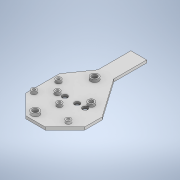
# Autodesk Inventor part: Część1
Saved by Autodesk Inventor 2020 (Build 240168000, 168)
## iProperties
Created: 2019-04-24
Part Number: Część1
Material: Ogólny
Document SubType Name: Modeling
Designer: atmat
Density: 1 g/cm^3
Appearance: Domyślna
Author: atmat
Autodesk Inventor part; units mm, degrees
ref_plane "YZ Plane" through (0, 0, 0) normal (1, 0, 0) x (0, 1, 0)
ref_plane "XZ Plane" through (0, 0, 0) normal (0, 1, 0) x (-1, 0, 0)
sketch "Szkic1" plane through (0, 0, 0) normal (0, 1, 0) x (-1, 0, 0)
  circle A0 centre (0, 22.5) radius 2
  circle A1 centre (0, -22.5) radius 2
  circle A2 centre (0, 22.5) radius 11.25 construction
  circle A3 centre (0, -22.5) radius 11.25 construction
  circle A4 centre (0, 0) radius 11.25
  circle A5 centre (-15.3043, -4.6667) radius 4.75 construction
  circle A6 centre (-15.3043, -4.6667) radius 12.25 construction
  circle A7 centre (-18.2464, 15.6211) radius 8.25 construction
  circle A8 centre (-18.2464, 15.6211) radius 1
  circle A9 centre (-15.3043, -4.6667) radius 1.5
  line L0 (17, 55) -> (-27.5543, 55)
  line L1 (-27.5543, 55) -> (-27.5543, -55)
  line L2 (-27.5543, -55) -> (17, -55)
  line L3 (17, -55) -> (17, 55)
  circle A10 centre (0, 22.5) radius 17 construction
  circle A11 centre (0, -22.5) radius 17 construction
  circle A12 centre (0, 0) radius 14.5 construction
  line L4 (12.5, 7.3485) -> (12.5, -7.3485) construction
  line L5 (-12.5, 7.3485) -> (-12.5, -7.3485) construction
  circle A13 centre (12.0332, -7.1556) radius 8.25 construction
  circle A14 centre (12.0332, -7.1556) radius 2.75 construction
  circle A15 centre (14.255, 9.1942) radius 8.25 construction
  circle A16 centre (14.255, 9.1942) radius 1
  circle A17 centre (12.0332, -7.1556) radius 1
  circle A18 centre (-3.8336, 8) radius 8.25 construction
  circle A19 centre (-3.8336, 8) radius 1
  circle A20 centre (-3.8336, 8) radius 2.75 construction
  circle A21 centre (4.6517, 1) radius 8.25 construction
  circle A22 centre (4.6517, 1) radius 1
  circle A23 centre (4.6517, 1) radius 2.75 construction
  line L6 (-27.5543, -0.6454) -> (-7, -30)
  line L7 (-7, -30) -> (-7, -64)
  line L8 (-7, -64) -> (5, -64)
  line L9 (5, -64) -> (5, -30)
  line L10 (5, -30) -> (17, -12.8622)
  line L11 (17, 12.5) -> (2, 27.5)
  line L12 (2, 27.5) -> (-12.5543, 27.5)
  line L13 (-12.5543, 27.5) -> (-27.5543, 12.5)
  circle A24 centre (0, 0) radius 2
  circle A25 centre (-9.3126, 0) radius 11.25 construction
  circle A26 centre (-9.3126, 0) radius 2
  circle A27 centre (-15.3227, 0) radius 11.25 construction
  circle A28 centre (-15.3227, 0) radius 2
  point P0 (-7, -55)
  point P1 (5, -55)
  dimension "d0" = 4
  dimension "d1" = 4
  dimension "d2" = 22.5
  dimension "d3" = 22.5
  dimension "d4" = 22.5
  dimension "d5" = 22.5
  dimension "d6" = 22.5
  dimension "d7" = 9.5
  dimension "d8" = 24.5
  dimension "d9" = 16.5
  dimension "d10" = 2
  dimension "d11" = 3
  dimension "d12" = 34
  dimension "d13" = 34
  dimension "d14" = 29
  dimension "d15" = 25
  dimension "d16" = 17
  dimension "d17" = 55
  dimension "d18" = 110
  dimension "d21" = 16.5
  dimension "d22" = 5.5
  dimension "d23" = 16.5
  dimension "d24" = 45
  dimension "d26" = 2
  dimension "d27" = 2
  dimension "d28" = 16.5
  dimension "d29" = 2
  dimension "d30" = 5.5
  dimension "d33" = 16.5
  dimension "d34" = 27.5543
  dimension "d35" = 2
  dimension "d36" = 5.5
  dimension "d39" = 12
  dimension "d40" = 12
  dimension "d41" = 0
  dimension "d42" = 9
  dimension "d43" = 145
  dimension "d44" = 145
  dimension "d45" = 25
  dimension "d46" = 45
  dimension "d47" = 45
  dimension "d48" = 15
  dimension "d49" = 5
  dimension "d50" = 0
  dimension "d63" = 1
  dimension "d64" = 8
  dimension "d65" = 4
  dimension "d66" = 22.5
  dimension "d67" = 0
  dimension "d68" = 4
  dimension "d69" = 22.5
  dimension "d70" = 0
  dimension "d71" = 4
  constraints: 29 centre point, 28 end point, 19 coincident, 13 tangent, 4 parallel, 4 point on circle, 4 point on line, 3 perpendicular, 2 horizontal, 2 vertical
  measures "d0" diameter of A0
  measures "d1" diameter of A1
  measures "d2" distance of point (0, 0) A0.centre
  measures "d3" distance of point (0, 0) A1.centre
  measures "d4" diameter of A2
  measures "d5" diameter of A3
  measures "d6" diameter of A4
  measures "d7" diameter of A5
  measures "d8" diameter of A6
  measures "d9" diameter of A7
  measures "d10" diameter of A8
  measures "d11" diameter of A9
  measures "d12" diameter of A10
  measures "d13" diameter of A11
  measures "d14" diameter of A12
  measures "d15" distance between parallel lines of L4 L5
  measures "d16" distance from line of L3 A4.centre
  measures "d17" distance from line of point (0, 0) L0
  measures "d18" distance between parallel lines of L2 L0
  measures "d21" diameter of A13
  measures "d22" diameter of A14
  measures "d23" diameter of A15
  measures "d24" distance of A0.centre A1.centre
  measures "d26" diameter of A16
  measures "d27" diameter of A17
  measures "d28" diameter of A18
  measures "d29" diameter of A19
  measures "d30" diameter of A20
  measures "d33" diameter of A21
  measures "d34" distance from line of L1 A1.centre
  measures "d35" diameter of A22
  measures "d36" diameter of A23
  measures "d39" distance between parallel lines of L3 L9
  measures "d40" distance between parallel lines of L9 L7
  measures "d41" vertical distance of L6.end L9.end
  measures "d42" distance between parallel lines of L2 L8
  measures "d43" angle of L9 L10
  measures "d44" angle of L7 L6
  measures "d45" distance from line of L2 L9.end
  measures "d46" angle of L3 L11
  measures "d47" angle of L1 L13
  measures "d48" distance from line of L3 L11.end
  measures "d49" distance from line of A0.centre L12
  measures "d50" vertical distance of L11.start L13.end
  measures "d63" vertical distance of A21.centre point (0, 0)
  measures "d64" vertical distance of A18.centre point (0, 0)
  measures "d65" diameter of A24
  measures "d66" diameter of A25
  measures "d67" vertical distance of point (0, 0) A25.centre
  measures "d68" diameter of A26
  measures "d69" diameter of A27
  measures "d70" vertical distance of A24.centre A27.centre
  measures "d71" diameter of A28
ref_plane "Płaszczyzna konstrukcyjna1" through (0, 2, 0) normal (0, 1, 0) x (1, 0, 0)
sketch "Szkic2" plane through (0, 2, 0) normal (0, 1, 0) x (1, 0, 0)
  circle A0 centre (0, -22.5) radius 2
  circle A1 centre (-14.255, -9.1942) radius 1
  circle A2 centre (3.8336, -8) radius 1
  circle A3 centre (-4.6517, -1) radius 1
  circle A4 centre (15.3043, 4.6667) radius 1.5
  circle A5 centre (0, 22.5) radius 2
  circle A6 centre (-12.0332, 7.1556) radius 1
  circle A7 centre (18.2464, -15.6211) radius 1
  circle A8 centre (0, -22.5) radius 2 projected
  circle A9 centre (-14.255, -9.1942) radius 1 projected
  circle A10 centre (3.8336, -8) radius 1 projected
  circle A11 centre (-4.6517, -1) radius 1 projected
  circle A12 centre (15.3043, 4.6667) radius 1.5 projected
  circle A13 centre (18.2464, -15.6211) radius 1 projected
  circle A14 centre (0, 22.5) radius 2 projected
  circle A15 centre (-12.0332, 7.1556) radius 1 projected
  circle A16 centre (0, -22.5) radius 3
  circle A17 centre (-14.255, -9.1942) radius 2
  circle A18 centre (3.8336, -8) radius 2
  circle A19 centre (-4.6517, -1) radius 2
  circle A20 centre (18.2464, -15.6211) radius 2
  circle A21 centre (15.3043, 4.6667) radius 2.5
  circle A22 centre (0, 22.5) radius 3
  circle A23 centre (-12.0332, 7.1556) radius 2
  point P0 (0, 0)
  dimension "d53" = 1
  dimension "d54" = 1
  dimension "d55" = 1
  dimension "d56" = 1
  dimension "d57" = 1
  dimension "d58" = 1
  dimension "d59" = 1
  dimension "d60" = 1
  constraints: 16 centre point, 16 concentric, 8 coincident
  measures "d53" radial gap between concentric circles of A0 A16
  measures "d54" radial gap between concentric circles of A17 A1
  measures "d55" radial gap between concentric circles of A18 A2
  measures "d56" radial gap between concentric circles of A19 A3
  measures "d57" radial gap between concentric circles of A20 A7
  measures "d58" radial gap between concentric circles of A21 A4
  measures "d59" radial gap between concentric circles of A22 A5
  measures "d60" radial gap between concentric circles of A23 A15
extrude "Wyciągnięcie proste6" add sketch "Szkic1" along normal blind 2 contours A4 A26 | L3 L10 L9 L2 L7 L6 L1 L13 L12 L11 picked at (-5.8126, -3.4695)
extrude "Wyciągnięcie proste7" add sketch "Szkic2" along normal blind 2
